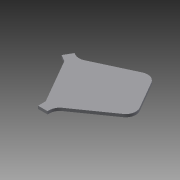
# Autodesk Inventor part: brazos
Saved by Autodesk Inventor 2015 (Build 190159000, 159)
## iProperties
Created: 2017-10-02
Part Number: brazos
Material: Generic
Document SubType Name: Modeling
Designer: macbook
Density: 1 g/cm^3
Appearance: Default
Author: macbook
Autodesk Inventor part; units mm, degrees
ref_plane "YZ Plane" through (0, 0, 0) normal (1, 0, 0) x (0, 1, 0)
ref_plane "XZ Plane" through (0, 0, 0) normal (0, 1, 0) x (-1, 0, 0)
ref_plane "XY Plane" through (0, 0, 0) normal (0, 0, 1) x (1, 0, 0)
sketch "Sketch1" plane through (0, 0, 0) normal (0, 0, 1) x (1, 0, 0)
  arc A0 (20, 100) -> (18.5818, 85) centre (115.8042, 83.3748) ccw
  arc A1 (-53.6995, 210.1948) -> (-40, 203.923) centre (-6.4957, 295.2045) ccw
  line L0 (-10, 117.3205) -> (0, 100)
  line L1 (-40, 169.282) -> (-50, 186.6025)
  line L2 (0, 100) -> (0, 85)
  line L3 (0, 85) -> (18.5818, 85)
  line L4 (-10, 117.3205) -> (-40, 169.282)
  line L5 (-50, 186.6025) -> (-62.9904, 194.1025)
  line L6 (-62.9904, 194.1025) -> (-53.6995, 210.1948)
  line L7 (87.5833, 208.3013) -> (62.5833, 251.6025)
  line L8 (87.5833, 208.3013) -> (112.5833, 165)
  line L9 (-40, 203.923) -> (62.5833, 251.6025)
  line L10 (20, 100) -> (112.5833, 165)
  dimension "d14" = 15
  dimension "d47" = 15
  dimension "d49" = 50
  dimension "d50" = 50
  constraints: 22 end point, 4 point on circle, 2 centre point, 2 collinear, 1 horizontal, 1 vertical
  measures "d14" distance of L2.end L0.end
  measures "d47" distance of L1.end L5.end
  measures "d49" distance of L7.start L7.end
  measures "d50" distance of L7.start L8.end
extrude "Extrusion4" add sketch "Sketch1" along normal blind 5.5
fillet "Fillet1" radius 20 2 edges at (112.5833, 165, 2.75) (62.5833, 251.6025, 2.75)
fillet "Fillet2" radius 20 2 edges at (20, 100, 2.75) (-40, 203.923, 2.75)
body "Solid3"
